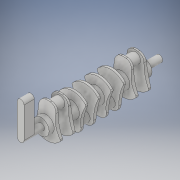
# Autodesk Inventor part: Crankshaft
Saved by Autodesk Inventor 2018 (Build 220112000, 112)
## iProperties
Created: 2019-08-26
Part Number: Crankshaft
Material: Generic
Document SubType Name: Modeling
Designer: 871357
Density: 1 g/cm^3
Appearance: Default
Author: 871357
Autodesk Inventor part; units mm, degrees
sketch "Sketch1" plane through (0, 0, 0) normal (0, 0, 1) x (1, 0, 0)
  circle A0 centre (0, 0) radius 12.7
  dimension "d0" = 25.4
  constraints: 1 centre point, 1 coincident
  measures "d0" diameter of A0
extrude "Extrusion1" add sketch "Sketch1" against normal blind 50.8
sketch "Sketch2" plane through (0, 0, -50.8) normal (0, 0, -1) x (-1, 0, 0)
  circle A0 centre (0, 0) radius 29.972
  dimension "d3" = 59.944
  constraints: 1 centre point, 1 coincident
  measures "d3" diameter of A0
extrude "Extrusion2" add sketch "Sketch2" along normal blind 25.4
ref_plane "Work Plane1" through (0, 0, -82.55) normal (0, 0, -1) x (-1, 0, 0)
ref_plane "Work Plane2" through (0, 0, -88.9) normal (0, 0, -1) x (-1, 0, 0)
sketch "Sketch3" plane through (0, 0, -82.55) normal (0, 0, -1) x (-1, 0, 0)
  circle A0 centre (0, 0) radius 72.39
  dimension "d8" = 144.78
  constraints: 1 centre point, 1 coincident
  measures "d8" diameter of A0
loft "Loft1" add profiles "Sketch3" section 1 edges at (29.972, 0, -76.2)
extrude "Extrusion3" add sketch "Sketch3" along normal blind 6.35
sketch "Sketch4" plane through (0, 0, -88.9) normal (0, 0, -1) x (-1, 0, 0)
  circle A0 centre (0, 46.99) radius 19.05
  point P0 (0, 0)
  dimension "d15" = 38.1
  dimension "d16" = 46.99
  constraints: 1 centre point
  measures "d15" diameter of A0
  measures "d16" distance of point (0, 0) A0.centre
extrude "Extrusion4" add sketch "Sketch4" along normal blind 38.1
sketch "Sketch5" plane through (0, 46.99, -127) normal (0, 0, -1) x (-1, 0, 0)
  circle A0 centre (0, -46.99) radius 72.39
  constraints: 1 centre point, 1 coincident
extrude "Extrusion5" add sketch "Sketch5" along normal blind 6.35
ref_plane "Work Plane3" through (0, 0, -139.7) normal (0, 0, -1) x (-1, 0, 0)
sketch "Sketch6" plane through (0, 0, -139.7) normal (0, 0, -1) x (-1, 0, 0)
  circle A0 centre (0, 0) radius 29.972 projected
loft "Loft2" add profiles "Sketch6" section 2 edges at (72.39, 0, -133.35)
extrude "Extrusion6" add sketch "Sketch6" along normal blind 30.48
ref_plane "Work Plane4" through (0, 0, -176.53) normal (0, 0, -1) x (-1, 0, 0)
sketch "Sketch7" plane through (0, 0, -176.53) normal (0, 0, -1) x (-1, 0, 0)
  circle A0 centre (0, 0) radius 72.39
  dimension "d29" = 144.78
  constraints: 1 centre point, 1 coincident
  measures "d29" diameter of A0
loft "Loft3" add profiles "Sketch7" section 1 edges at (29.972, 0, -170.18)
extrude "Extrusion7" add sketch "Sketch7" along normal blind 6.35
sketch "Sketch8" plane through (0, 0, -182.88) normal (0, 0, -1) x (-1, 0, 0)
  circle A0 centre (0, -46.99) radius 19.05
  point P0 (0, 0)
  dimension "d36" = 38.1
  dimension "d37" = 46.99
  constraints: 1 centre point
  measures "d36" diameter of A0
  measures "d37" distance of point (0, 0) A0.centre
extrude "Extrusion8" add sketch "Sketch8" along normal blind 38.1
sketch "Sketch9" plane through (0, 0, -88.9) normal (0, 0, -1) x (-1, 0, 0)
  circle A0 centre (0, 46.99) radius 19.05 construction
  circle A1 centre (0, 46.99) radius 19.05 construction
  line L0 (0, 71.4265) -> (0, 74.6163) construction
  circle A2 centre (0, 0) radius 72.39 construction
  arc A3 (-86.36, -80.01) -> (-33.02, 64.4204) centre (-196.6988, 42.8043) ccw
  arc A4 (-33.02, 64.4204) -> (-86.36, -80.01) centre (-34.8694, -16.9614) ccw
  arc A5 (33.02, 64.4204) -> (86.36, -80.01) centre (196.6988, 42.8043) ccw
  arc A6 (86.36, -80.01) -> (33.02, 64.4204) centre (34.8694, -16.9614) ccw
  point P0 (0, 72.39)
  point P1 (0, 72.39)
  dimension "d42" = 33.02
  dimension "d43" = 165.1
  dimension "d44" = 152.4
  dimension "d45" = 7.9696
  dimension "d59" = 86.36
  dimension "d60" = 86.36
  constraints: 9 point on circle, 4 centre point, 4 symmetric about line, 2 end point, 2 vertical alignment, 1 vertical, 2 other
  measures "d42" horizontal distance of A2.start A3.end
  measures "d43" radius of A3
  measures "d44" vertical distance of A2.start A3.start
  measures "d45" vertical distance of A2.start A3.end
  measures "d59" horizontal distance of A2.start A3.start
  measures "d60" horizontal distance of A6.start A2.start
extrude "Extrusion9" cut sketch "Sketch9" along normal mid plane 114.3
fillet "Fillet1" radius 25.4 4 edges at (33.02, 64.4204, -85.725) (-33.02, 64.4204, -85.725) (-33.02, 64.4204, -130.175) (33.02, 64.4204, -130.175)
sketch "Sketch10" plane through (0, -46.99, -220.98) normal (0, 0, -1) x (-1, 0, 0)
  circle A0 centre (0, 46.99) radius 72.39
  constraints: 1 centre point, 1 coincident
extrude "Extrusion10" add sketch "Sketch10" along normal blind 6.35
ref_plane "Work Plane5" through (0, 0, -233.68) normal (0, 0, -1) x (-1, 0, 0)
sketch "Sketch11" plane through (0, 0, -233.68) normal (0, 0, -1) x (-1, 0, 0)
  circle A0 centre (0, 0) radius 29.972 projected
  circle A1 centre (0, 0) radius 29.972 projected
loft "Loft4" add profiles "Sketch11" section 1 edges at (72.39, 0, -227.33)
sketch "Sketch12" plane through (0, 0, -233.68) normal (0, 0, -1) x (-1, 0, 0)
  circle A0 centre (0, 0) radius 29.972 projected
extrude "Extrusion11" add sketch "Sketch12" along normal blind 15.24
sketch "Sketch13" plane through (0, 0, -233.68) normal (0, 0, -1) x (-1, 0, 0)
  arc A0 (86.36, 80.01) -> (33.0318, -64.4144) centre (196.71, -42.7942) ccw
  circle A1 centre (0, 0) radius 72.39 construction
  circle A2 centre (0, 0) radius 29.972 construction
  circle A3 centre (0, 0) radius 72.39 construction
  arc A4 (33.0318, -64.4144) -> (86.36, 80.01) centre (-0.0621, 29.8633) ccw
  line L0 (-0.0621, 61.8194) -> (-0.0621, 43.4287) construction
  arc A5 (-33.1561, -64.4144) -> (-86.4843, 80.01) centre (-196.8343, -42.7942) ccw
  arc A6 (-86.4843, 80.01) -> (-33.1561, -64.4144) centre (-0.0621, 29.8633) ccw
  point P0 (0, -72.39)
  dimension "d56" = 165.1
  dimension "d57" = 7.9756
  dimension "d58" = 152.4
  dimension "d61" = 86.36
  dimension "d62" = 0
  constraints: 9 point on circle, 4 centre point, 3 symmetric about line, 2 end point, 1 vertical, 4 other
  measures "d56" radius of A0
  measures "d57" vertical distance of A3.end A0.end
  measures "d58" vertical distance of A0.start A3.end
  measures "d61" horizontal distance of A3.end A0.start
  measures "d62" horizontal distance of point (0, 0) A3.end
extrude "Extrusion12" cut sketch "Sketch13" against normal blind 76.2
fillet "Fillet2" radius 25.4 4 edges at (-33.0318, -64.4144, -224.155) (33.1482, -64.3546, -224.155) (33.1482, -64.3546, -179.705) (-33.0318, -64.4144, -179.705)
fillet "Fillet3" radius 6.35 8 edges at (56.8759, 44.7822, -224.155) (56.8759, 44.7822, -179.705) (-56.8066, 44.8701, -224.155) (-56.8066, 44.8701, -179.705) (56.8038, -44.8735, -85.725) (56.8038, -44.8735, -130.175) (-56.8038, -44.8735, -130.175) (-56.8038, -44.8735, -85.725)
mirror "Mirror1" about plane through (0, 0, -248.92) normal (0, 0, -1) of "Extrusion1", "Extrusion2", "Extrusion9", "Extrusion4", "Extrusion6", "Extrusion5", "Extrusion7", "Extrusion12", "Extrusion11", "Extrusion10", "Extrusion8", "Loft2", "Extrusion3", "Fillet1", "Loft1", "Loft3", "Loft4", "Fillet2", "Fillet3"
sketch "Sketch14" plane through (0, 0, -50.8) normal (0, 0, 1) x (1, 0, 0)
  circle A0 centre (0, 0) radius 29.972 projected
  circle A1 centre (0, 0) radius 12.7 projected
extrude "Extrusion13" cut sketch "Sketch14" against normal blind 6.35
ref_plane "Work Plane8" through (0, 0, -248.92) normal (0, 0, 1) x (1, 0, 0)
mirror "Mirror2" about plane through (0, 0, -248.92) normal (0, 0, 1) of "Extrusion13"
sketch "Sketch15" plane through (0, 0, -88.9) normal (0, 0, -1) x (-1, 0, 0)
  arc A0 (-53.7175, -48.5257) -> (53.7175, -48.5257) centre (0, 0) ccw construction
  arc A1 (9.607, 71.7497) -> (-9.607, 71.7497) centre (0, 0) ccw construction
  circle A2 centre (0, 0) radius 29.972 construction
  arc A3 (-47.1215, -36.2154) -> (47.1213, -36.2157) centre (0, 6.35) ccw
  line L0 (-49.954, -32.8526) -> (49.954, -32.8526) construction
  line L1 (-49.954, -32.8526) -> (49.954, -32.8526) construction
  circle A4 centre (0, 0) radius 12.7 projected
  arc A5 (-48.1241, -29.1904) -> (-44.9888, -22.3269) centre (-198.3176, 43.5679) ccw
  arc A6 (-48.1241, -29.1904) -> (-47.1215, -36.2154) centre (-42.4094, -31.9588) ccw
  arc A7 (43.3498, -18.3684) -> (48.1239, -29.1907) centre (197.3841, 43.1168) ccw
  arc A8 (47.1213, -36.2157) -> (48.1239, -29.1907) centre (42.4091, -31.9591) ccw
  line L2 (-44.9888, -22.3269) -> (-60.8075, -34.0428)
  line L3 (-60.8075, -34.0428) -> (-60.8075, -66.4653)
  line L4 (-60.8075, -66.4653) -> (17.6144, -89.161)
  line L5 (17.6144, -89.161) -> (66.588, -58.8605)
  line L6 (66.588, -58.8605) -> (66.588, -19.4526)
  line L7 (66.588, -19.4526) -> (43.3498, -18.3684)
  dimension "d69" = 0
  dimension "d70" = 63.5
  dimension "d71" = 6.35
  dimension "d72" = 6.35
  dimension "d73" = 6.35
  constraints: 16 end point, 14 point on circle, 5 centre point, 4 tangent, 1 collinear, 1 horizontal, 1 parallel, 1 vertical, 10 other
  measures "d69" distance between parallel lines of L0 L1
  measures "d70" radius of A3
  measures "d71" distance of A4.centre A3.centre
  measures "d72" radius of A6
  measures "d73" radius of A8
extrude "Extrusion14" cut sketch "Sketch15" along normal mid plane 101.6 contours A3 A8 A7 L7 L6 L5 L4 L3 L2 A5 A6
ref_plane "Work Plane9" through (0, 0, -201.93) normal (0, 0, -1) x (-1, 0, 0)
sketch "Sketch16" plane through (0, 0, -201.93) normal (0, 0, -1) x (-1, 0, 0)
  arc A0 (-31.7665, -46.0545) -> (-54.5561, 40.9608) centre (-196.8343, -42.7942) ccw construction
  arc A1 (54.4791, 41.0411) -> (31.6425, -46.069) centre (196.71, -42.7942) ccw construction
  arc A2 (47.1081, 36.1614) -> (-47.2324, 36.1614) centre (-0.0621, -6.35) ccw
  line L0 (-50.0573, 32.8002) -> (49.933, 32.8002) construction
  line L1 (-50.0573, 32.8002) -> (49.933, 32.8002) construction
  arc A3 (-44.2179, 20.1837) -> (-48.2309, 29.1434) centre (-196.8343, -42.7942) ccw
  arc A4 (48.1066, 29.1434) -> (43.269, 18.1473) centre (196.71, -42.7942) ccw
  arc A5 (48.1066, 29.1434) -> (47.1081, 36.1614) centre (42.3911, 31.9102) ccw
  arc A6 (-47.2324, 36.1614) -> (-48.2309, 29.1434) centre (-42.5154, 31.9102) ccw
  line L2 (-44.2179, 20.1837) -> (-74.0629, 23.0135)
  line L3 (-74.0629, 23.0135) -> (-68.3325, 83.4505)
  line L4 (-68.3325, 83.4505) -> (6.0963, 95.9365)
  line L5 (6.0963, 95.9365) -> (79.414, 74.7622)
  line L6 (79.414, 74.7622) -> (76.0197, 16.2475)
  line L7 (76.0197, 16.2475) -> (43.269, 18.1473)
  point P0 (0, 0)
  dimension "d76" = 0
  dimension "d77" = 63.5
  dimension "d78" = 6.35
  dimension "d79" = 6.35
  constraints: 18 point on circle, 16 end point, 5 centre point, 4 tangent, 3 equal radius, 2 perpendicular, 1 collinear, 1 horizontal
  measures "d76" distance between parallel lines of L0 L1
  measures "d77" radius of A2
  measures "d78" vertical distance of point (0, 0) A2.centre
  measures "d79" radius of A5
extrude "Extrusion15" cut sketch "Sketch16" along normal blind 127
extrude "Extrusion16" cut sketch "Sketch16" against normal blind 50.8
sketch "Sketch17" plane through (0, 0, -408.94) normal (0, 0, 1) x (1, 0, 0)
  arc A0 (-47.1215, -36.2155) -> (47.1212, -36.2158) centre (0, 6.35) ccw
  line L0 (49.954, -32.8526) -> (-49.954, -32.8526) construction
  line L1 (49.954, -32.8526) -> (149.862, -32.8526) construction
  circle A1 centre (0, 0) radius 12.7 construction
  arc A2 (41.6005, -13.7865) -> (48.1238, -29.1907) centre (197.1114, 42.9851) ccw
  arc A3 (-48.1241, -29.1906) -> (-44.2439, -20.5638) centre (-197.8581, 43.343) ccw
  arc A4 (47.1212, -36.2158) -> (48.1238, -29.1907) centre (42.4091, -31.9592) ccw
  arc A5 (-48.1241, -29.1906) -> (-47.1215, -36.2155) centre (-42.4093, -31.9589) ccw
  line L2 (-44.2439, -20.5638) -> (-58.4356, -24.9048)
  line L3 (-58.4356, -24.9048) -> (-64.584, -79.2035)
  line L4 (-64.584, -79.2035) -> (-4.1613, -94.6133)
  line L5 (-4.1613, -94.6133) -> (44.6674, -91.5744)
  line L6 (44.6674, -91.5744) -> (60.5833, -68.5737)
  line L7 (60.5833, -68.5737) -> (60.5833, -13.7865)
  line L8 (60.5833, -13.7865) -> (41.6005, -13.7865)
  dimension "d84" = 180
  dimension "d85" = 63.5
  dimension "d86" = 6.35
  dimension "d87" = 6.35
  constraints: 18 end point, 14 point on circle, 5 centre point, 4 tangent, 1 collinear, 1 equal radius, 1 horizontal, 1 perpendicular, 1 vertical, 6 other
  measures "d84" angle of L0 L1
  measures "d85" radius of A0
  measures "d86" distance of A1.centre A0.centre
  measures "d87" radius of A4
extrude "Extrusion17" cut sketch "Sketch17" along normal mid plane 101.6
sketch "Sketch18" plane through (0, 0, 0) normal (0, 0, 1) x (1, 0, 0)
  circle A0 centre (0, 0) radius 12.7 construction
  line L0 (-12.7, 0) -> (12.7, 0)
  line L1 (12.7, 0) -> (12.7, 127)
  line L2 (12.7, 127) -> (-12.7, 127)
  line L3 (-12.7, 127) -> (-12.7, 0)
  dimension "d90" = 127
  constraints: 8 end point, 2 parallel, 1 horizontal, 1 horizontal alignment, 1 perpendicular, 1 other
  measures "d90" distance of L1.end L0.end
extrude "Extrusion18" add sketch "Sketch18" along normal mid plane 38.1
sketch "Sketch19" plane through (0, 0, 0) normal (0, 0, 1) x (1, 0, 0)
  line L0 (12.7, 0) -> (-12.7, 0) projected
  arc A0 (-12.7, 0) -> (12.7, 0) centre (0, 0) ccw projected
extrude "Extrusion19" add sketch "Sketch19" along normal up to surface (19.05 mm away)
fillet "Fillet4" radius 12.7 2 edges at (12.7, 127, 0) (-12.7, 127, 0)
ref_plane "Work Plane6" through (0, 0, -408.94) normal (0, 0, -1) x (-1, 0, 0)
ref_plane "Work Plane7" through (0, 0, -358.14) normal (0, 0, -1) x (-1, 0, 0)
body "Solid1"
